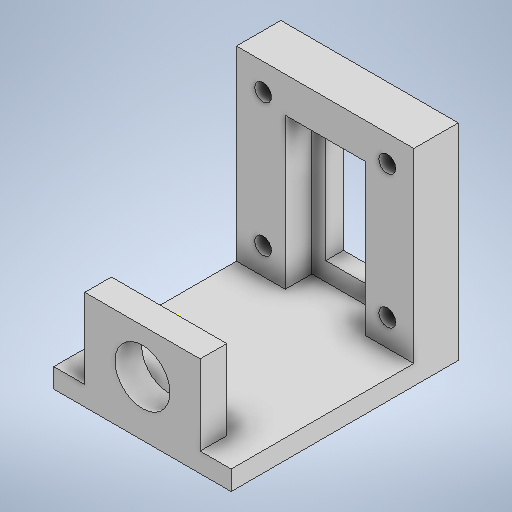
# Autodesk Inventor part: laser_krabicka2
Saved by Autodesk Inventor 2025.2 (Build 292293000, 293)
## iProperties
Created: 2025-03-31
Part Number: laser_krabicka2
Material: Všeobecné
Document SubType Name: Modeling
Designer: jakub
Density: 1 g/cm^3
Appearance: Výchozí
Author: jakub
## iProperties of the stored document laser_krabicka2_3D tisk.ipt
Created: 2025-03-31
Part Number: laser_krabicka2_3D tisk
Material: Všeobecné
Document SubType Name: Modeling
Designer: jakub
Density: 1 g/cm^3
Appearance: Výchozí
Author: jakub
Autodesk Inventor part; units mm, degrees
ref_plane "YZ Plane" through (0, 0, 0) normal (1, 0, 0) x (0, 1, 0)
ref_plane "XZ Plane" through (0, 0, 0) normal (0, 1, 0) x (-1, 0, 0)
sketch "Náčrt1" plane through (0, 0, 0) normal (0, 0, 1) x (1, 0, 0)
  line L0 (0, 12.6) -> (0, -12.6) projected
  line L1 (-12.6, 0) -> (12.6, 0) projected
  line L2 (-9, 9) -> (9, 9)
  line L3 (9, 9) -> (9, -9)
  line L4 (9, -9) -> (-9, -9)
  line L5 (-9, -9) -> (-9, 9)
  point P0 (0, 0)
  dimension "d0" = 18
  dimension "d1" = 18
  constraints: 8 end point, 2 parallel, 1 horizontal, 1 perpendicular, 2 other
  measures "d0" distance between parallel lines of L5 L3
  measures "d1" distance between parallel lines of L4 L2
extrude "Vysunutí1" add sketch "Náčrt1" against normal blind 20
sketch "Náčrt2" plane through (-9, 9, 0) normal (0, 1, 0) x (1, 0, 0)
  line L0 (18, 0) -> (0, 0) projected
  line L1 (18, 0) -> (18, 20) projected
  line L2 (0, 20) -> (18, 20) projected
  line L3 (0, 0) -> (0, 20) projected
  line L4 (1.3, 16.6) -> (1.3, 3)
  line L5 (1.3, 3) -> (16.7, 3)
  line L6 (16.7, 3) -> (16.7, 16.6)
  line L7 (16.7, 16.6) -> (1.3, 16.6)
  point P0 (9, 0)
  dimension "d4" = 3.4
  dimension "d5" = 3
  dimension "d6" = 1.3
  dimension "d7" = 1.3
  constraints: 8 end point, 3 perpendicular, 1 vertical
  measures "d4" distance between parallel lines of L2 L7
  measures "d5" distance between parallel lines of L0 L5
  measures "d6" distance between parallel lines of L6 L1
  measures "d7" distance between parallel lines of L3 L4
sketch "Náčrt3" plane through (0, 0, 0) normal (0, 0, 1) x (1, 0, 0)
  point P0 (0, 0)
extrude "Vysunutí2" cut sketch "Náčrt2" against normal blind 17 contours L7 L6 L5 L4
sketch "Náčrt4" plane through (0, 0, 0) normal (0, 0, 1) x (1, 0, 0)
  line L0 (0, 12.6) -> (0, -12.6) projected
  line L1 (-12.6, 0) -> (12.6, 0) projected
  circle A0 centre (0, -4) radius 3.1
  line L2 (-9, -9) -> (9, -9) projected
  point P0 (0, 0)
  dimension "d10" = 6.2
  dimension "d11" = 5
  constraints: 1 centre point, 1 point on line
  measures "d10" diameter of A0
  measures "d11" distance from line of L2 A0.centre
extrude "Vysunutí3" cut sketch "Náčrt4" against normal blind 3
sketch "Náčrt5" plane through (-9, 9, 0) normal (0, 1, 0) x (1, 0, 0)
  line L0 (1.3, 3) -> (1.3, 16.6) projected
  line L1 (1.3, 16.6) -> (16.7, 16.6) projected
  line L2 (16.7, 3) -> (1.3, 3) projected
  line L3 (16.7, 16.6) -> (16.7, 3) projected
  line L4 (1.3, 16.6) -> (16.7, 16.6) projected
  line L5 (1.3, 3) -> (1.3, 16.6) projected
  line L6 (16.7, 16.6) -> (16.7, 3) projected
  line L7 (16.7, 16.6) -> (16.7, 3) projected
  line L8 (16.7, 3) -> (1.3, 3) projected
  line L9 (1.3, 3) -> (1.3, 16.6) projected
  line L10 (1.3, 16.6) -> (16.7, 16.6) projected
  line L11 (18, 0) -> (0, 0) projected
  line L12 (18, 0) -> (18, 20) projected
  line L13 (0, 20) -> (18, 20) projected
  line L14 (0, 0) -> (0, 20) projected
  line L15 (1.3, 16.6) -> (0, 16.6)
  line L16 (0, 0) -> (0, 20) projected
  line L17 (0, 16.6) -> (0, 0)
  line L18 (0, 0) -> (18, 0)
  line L19 (18, 0) -> (18, 16.6)
  line L20 (18, 0) -> (18, 20) projected
  line L21 (16.7, 16.6) -> (18, 16.6)
  line L22 (16.7, 16.6) -> (16.7, 3)
  line L23 (16.7, 3) -> (1.3, 3) projected
  line L24 (16.7, 3) -> (1.3, 3)
  line L25 (1.3, 3) -> (1.3, 16.6)
  line L26 (1.3, 3) -> (1.3, 16.6)
  point P0 (9, 0)
  constraints: 18 end point, 4 point on line, 2 collinear, 2 parallel, 2 perpendicular, 1 horizontal
extrude "Vysunutí4" cut sketch "Náčrt5" against normal blind 8 contours L2 L3 L21 L12 L11 L14 L15 L0
sketch "Náčrt6" plane through (0, 0, -20) normal (0, 0, -1) x (-1, 0, 0)
  line L0 (-9, -9) -> (9, -9) projected
  line L1 (9, -9) -> (9, 9) projected
  line L2 (9, 9) -> (-9, 9) projected
  line L3 (-9, 9) -> (-9, -9) projected
  line L4 (0, -12.6) -> (0, 12.6) projected
  line L5 (-12.6, 0) -> (12.6, 0) projected
  line L6 (-2.8665, 6.0827) -> (2.9335, 6.0827)
  line L7 (2.9335, 6.0827) -> (2.9335, -5.9173)
  line L8 (2.9335, -5.9173) -> (-2.8665, -5.9173)
  line L9 (-2.8665, -5.9173) -> (-2.8665, 6.0827)
  point P0 (0, 0)
  dimension "d16" = 5.8
  dimension "d17" = 12
  constraints: 8 end point, 2 parallel, 1 horizontal, 1 perpendicular
  measures "d16" distance between parallel lines of L9 L7
  measures "d17" distance between parallel lines of L8 L6
extrude "Vysunutí5" cut sketch "Náčrt6" against normal blind 8 contours L8 L9 L5 L4 | L4 L5 L7 L8 | L9 L6 L4 L5 | L4 L6 L7 L5
sketch "Náčrt13" plane through (9, -9, -20) normal (1, 0, 0) x (0, 0, -1)
  line L0 (-3.4, 10) -> (-20, 10) projected
  line L1 (-20, 0) -> (-20, 10) projected
  line L2 (-20, 0) -> (0, 0) projected
  line L3 (0, 18) -> (0, 0) projected
  line L4 (-3.4, 18) -> (0, 18) projected
  line L5 (-3.4, 18) -> (-3.4, 10) projected
  line L6 (-3.4, 1) -> (-17, 1) projected
  line L7 (-17, 1) -> (-3.4, 1) projected
  line L8 (-17, 10) -> (-3.4, 10) projected
  line L9 (-17, 1) -> (-17, 10)
  line L10 (-17, 8.1) -> (-17, 1.9) projected
  line L11 (-3.4, 1) -> (-3.4, 10)
  line L12 (-3.4, 1) -> (-17, 1)
  line L13 (-3.4, 10) -> (-17, 10)
  point P0 (-20, 9)
  constraints: 8 end point, 3 collinear, 1 parallel
extrude "Vysunutí11" cut sketch "Náčrt13" against normal blind 20 contours L11 L6 L9 L0
sketch "Náčrt14" plane through (0, 0, 0) normal (0, 0, 1) x (1, 0, 0)
  line L0 (9, 1) -> (-9, 1) projected
  line L1 (-9, 1) -> (-9, -9) projected
  line L2 (-9, -9) -> (9, -9) projected
  line L3 (9, -9) -> (9, 1) projected
  circle A0 centre (0, -4) radius 3.1 projected
  line L4 (2.8665, -5.9173) -> (-2.9335, -5.9173) projected
  line L5 (9, -8) -> (-9, -8) projected
  line L6 (9, -8) -> (-9, -8) projected
  line L7 (9, 1) -> (6.5, 1)
  line L8 (6.5, 1) -> (6.5, -8)
  line L9 (6.5, -8) -> (9, -8)
  line L10 (9, -8) -> (9, 1)
  line L11 (-9, 1) -> (-6.5, 1)
  line L12 (-6.5, 1) -> (-6.5, -8)
  line L13 (-6.5, -8) -> (-9, -8)
  line L14 (-9, -8) -> (-9, 1)
  point P0 (0, 0)
  dimension "d44" = 2.5
  dimension "d45" = 2.5
  constraints: 16 end point, 4 parallel, 2 horizontal, 2 perpendicular, 2 point on line
  measures "d44" distance between parallel lines of L8 L10
  measures "d45" distance between parallel lines of L1 L12
extrude "Vysunutí12" cut sketch "Náčrt14" against normal blind 5 contours L3 L5 L8 L0 | L12 L5 L1 L0
sketch "Náčrt15" plane through (-9, -9, 0) normal (0, -1, 0) x (1, 0, 0)
  line L0 (0, 0) -> (18, 0) projected
  line L1 (0, 0) -> (0, -20) projected
  line L2 (18, -20) -> (0, -20) projected
  line L3 (18, 0) -> (18, -20) projected
  line L4 (18, 0) -> (0, 0)
  line L5 (0, 0) -> (0, -20)
  line L6 (0, -20) -> (18, -20)
  line L7 (18, -20) -> (18, 0)
  point P0 (9, 0)
  constraints: 8 end point, 2 parallel, 1 horizontal, 1 perpendicular
extrude "Vysunutí13" add sketch "Náčrt15" along normal blind 1.2
sketch "Náčrt16" plane through (9, -8, -16.6) normal (1, 0, 0) x (0, 0, -1)
  line L0 (0, 0) -> (-16.6, 0) projected
  line L1 (-16.6, -2.2) -> (-16.6, 0) projected
  line L2 (3.4, -2.2) -> (-16.6, -2.2) projected
  line L3 (3.4, 17) -> (3.4, -2.2) projected
  line L4 (0, 17) -> (3.4, 17) projected
  line L5 (0, 17) -> (0, 0) projected
  line L6 (-16.6, 0) -> (3.4, 0)
  line L7 (3.4, 0) -> (3.4, -2.2)
  line L8 (3.4, -2.2) -> (-16.6, -2.2)
  line L9 (-16.6, -2.2) -> (-16.6, 0)
  line L10 (0, 17) -> (3.4, 17)
  line L11 (3.4, 17) -> (3.4, 0)
  line L12 (3.4, 0) -> (0, 0)
  line L13 (0, 0) -> (0, 17)
  point P0 (-16.6, 8)
  constraints: 16 end point, 4 parallel, 2 horizontal, 2 perpendicular
extrude "Vysunutí14" add sketch "Náčrt16" along normal blind 3
sketch "Náčrt17" plane through (-9, -8, -16.6) normal (-1, 0, 0) x (0, 0, 1)
  line L0 (16.6, 0) -> (0, 0) projected
  line L1 (0, 0) -> (0, 17) projected
  line L2 (0, 17) -> (-3.4, 17) projected
  line L3 (-3.4, 17) -> (-3.4, -2.2) projected
  line L4 (16.6, -2.2) -> (-3.4, -2.2) projected
  line L5 (16.6, 0) -> (16.6, -2.2) projected
  line L6 (-3.4, 17) -> (0, 17)
  line L7 (0, 17) -> (0, -2.2)
  line L8 (0, -2.2) -> (-3.4, -2.2)
  line L9 (-3.4, -2.2) -> (-3.4, 17)
  line L10 (16.6, 0) -> (0, 0)
  line L11 (0, 0) -> (0, -2.2)
  line L12 (0, -2.2) -> (16.6, -2.2)
  line L13 (16.6, -2.2) -> (16.6, 0)
  point P0 (16.6, 8)
  point P1 (0, -1.1)
  dimension "d52" = 3.4
  constraints: 16 end point, 4 parallel, 2 horizontal, 2 perpendicular, 1 midpoint, 1 point on line
  measures "d52" distance from line of L3 point (0, -1.1)
extrude "Vysunutí15" add sketch "Náčrt17" along normal blind 3
sketch "Náčrt18" plane through (0, 0, -20) normal (0, 0, -1) x (-1, 0, 0)
  line L0 (2.9335, 6.0827) -> (2.9335, -5.9173) projected
  line L1 (2.9335, -5.9173) -> (-2.8665, -5.9173) projected
  line L2 (-2.8665, -5.9173) -> (-2.8665, 6.0827) projected
  line L3 (-2.8665, 6.0827) -> (2.9335, 6.0827) projected
  line L4 (-12, 9) -> (12, 9) projected
  line L5 (-12, -10.2) -> (-12, 9) projected
  line L6 (-12, -10.2) -> (12, -10.2) projected
  line L7 (12, 9) -> (12, -10.2) projected
  line L8 (-12, 9) -> (12, 9)
  line L9 (12, 9) -> (12, -10.2)
  line L10 (12, -10.2) -> (-12, -10.2)
  line L11 (-12, -10.2) -> (-12, 9)
  line L12 (-2.8665, 6.0827) -> (2.9335, 6.0827)
  line L13 (2.9335, 6.0827) -> (2.9335, -5.9173)
  line L14 (2.9335, -5.9173) -> (-2.8665, -5.9173)
  line L15 (-2.8665, -5.9173) -> (-2.8665, 6.0827)
  point P0 (0, 0)
  constraints: 16 end point, 4 parallel, 2 horizontal, 2 perpendicular
extrude "Vysunutí16" add sketch "Náčrt18" along normal blind 1.6
sketch "Náčrt19" plane through (12, -8, -16.6) normal (0, 0, 1) x (1, 0, 0)
  line L0 (-24, 17) -> (0, 17) projected
  line L1 (0, 0) -> (-24, 0) projected
  line L2 (-16.5, 17) -> (-7.5, 17)
  line L3 (-7.5, 17) -> (-7.5, 0)
  line L4 (-7.5, 0) -> (-16.5, 0)
  line L5 (-16.5, 0) -> (-16.5, 17)
  line L6 (-14.9335, 2.0827) -> (-14.9335, 14.0827) projected
  line L7 (-14.9335, 14.0827) -> (-9.1335, 14.0827) projected
  line L8 (-9.1335, 14.0827) -> (-9.1335, 2.0827) projected
  line L9 (-9.1335, 2.0827) -> (-14.9335, 2.0827) projected
  line L10 (0, 0) -> (-24, 0) projected
  line L11 (0, 17) -> (0, 0) projected
  line L12 (-24, 17) -> (0, 17) projected
  line L13 (-24, 0) -> (-24, 17) projected
  line L14 (-12, 17) -> (-12, 0)
  line L15 (-16.5, 17) -> (-7.5, 17)
  line L16 (-16.5, 0) -> (-7.5, 0)
  point P0 (-12, 8)
  point P1 (-16.5, 0)
  dimension "d57" = 9
  constraints: 14 end point, 2 collinear, 2 midpoint, 2 parallel, 2 point on line, 1 horizontal, 1 perpendicular, 1 other
  measures "d57" distance between parallel lines of L5 L3
ref_plane "Pracovní rovina1" through (12, -8, -9.8) normal (0, 0, 1) x (1, 0, 0)
extrude "Vysunutí17" cut sketch "Náčrt19" against normal blind 3 contours L0 L14 L7 L6 L9 L1 L5 | L0 L3 L1 L14 L9 L8 L7
sketch "Náčrt20" plane through (-12, 9, -21.6) normal (0, 1, 0) x (1, 0, 0)
  line L0 (0, -5) -> (0, 0) projected
  line L1 (24, -5) -> (24, 0) projected
  line L2 (0, 0) -> (24, 0)
  line L3 (24, 0) -> (24, -5)
  line L4 (24, -5) -> (0, -5)
  line L5 (0, -5) -> (0, 0)
  point P0 (12, -21.6)
  constraints: 8 end point, 2 parallel, 1 horizontal, 1 perpendicular
extrude "Vysunutí18" add sketch "Náčrt20" along normal blind 4
sketch "Náčrt21" plane through (4.5, -8, -16.6) normal (0, 0, 1) x (1, 0, 0)
  line L0 (0, 17) -> (0, 0) projected
  line L1 (7.5, 0) -> (0, 0) projected
  line L2 (7.5, 0) -> (7.5, 21) projected
  line L3 (-16.5, 21) -> (7.5, 21) projected
  line L4 (-16.5, 0) -> (-16.5, 21) projected
  line L5 (-9, 0) -> (-16.5, 0) projected
  line L6 (-9, 0) -> (-9, 17) projected
  line L7 (-9, 17) -> (0, 17) projected
  circle A0 centre (-11.5, 18) radius 0.95
  circle A1 centre (2.5, 3) radius 0.95
  line L8 (7.5, 10.5) -> (-16.5, 10.5)
  circle A2 centre (2.5, 18) radius 0.95
  circle A3 centre (-11.5, 3) radius 0.95
  point P0 (-4.5, 8)
  dimension "d62" = 1.9
  dimension "d63" = 3
  dimension "d64" = 5
  dimension "d65" = 1.9
  dimension "d66" = 3
  dimension "d67" = 5
  constraints: 4 centre point, 2 end point, 2 midpoint, 2 symmetric about line, 2 other
  measures "d62" diameter of A0
  measures "d63" distance from line of A0.centre L3
  measures "d64" distance from line of L4 A0.centre
  measures "d65" diameter of A1
  measures "d66" distance from line of L1 A1.centre
  measures "d67" distance from line of L2 A1.centre
extrude "Vysunutí19" cut sketch "Náčrt21" against normal up to surface (5 mm away) contours A0 | A1 | A2 | A3
sketch "Náčrt22" plane through (-12, 13, -21.6) normal (0, 1, 0) x (1, 0, 0)
  line L0 (0, 0) -> (0, -5) projected
  line L1 (0, -5) -> (24, -5) projected
  line L2 (24, -5) -> (24, 0) projected
  line L3 (24, 0) -> (0, 0) projected
  line L4 (5.5, -21.6) -> (0, -21.6) projected
  line L5 (5.5, -21.6) -> (5.5, -18.6) projected
  line L6 (18.5, -18.6) -> (5.5, -18.6) projected
  line L7 (18.5, -21.6) -> (18.5, -18.6) projected
  line L8 (18.5, -21.6) -> (24, -21.6) projected
  line L9 (24, -5) -> (24, -21.6) projected
  line L10 (24, -5) -> (16.5, -5) projected
  line L11 (16.5, -5) -> (16.5, -2) projected
  line L12 (16.5, -2) -> (7.5, -2) projected
  line L13 (7.5, -5) -> (7.5, -2) projected
  line L14 (7.5, -5) -> (0, -5) projected
  line L15 (0, -21.6) -> (0, -5) projected
  line L16 (5.5, -18.6) -> (5.5, -21.6) projected
  line L17 (18.5, -21.6) -> (5.5, -21.6) projected
  line L18 (18.5, -21.6) -> (18.5, -18.6) projected
  line L19 (18.5, -18.6) -> (5.5, -18.6) projected
  line L20 (24, 0) -> (22, 0)
  line L21 (22, 0) -> (22, -21.6)
  line L22 (22, -21.6) -> (24, -21.6)
  line L23 (24, -21.6) -> (24, 0)
  line L24 (0, 0) -> (2, 0)
  line L25 (2, 0) -> (2, -21.6)
  line L26 (2, -21.6) -> (0, -21.6)
  line L27 (0, -21.6) -> (0, 0)
  point P0 (12, -21.6)
  dimension "d71" = 2
  dimension "d72" = 2
  constraints: 16 end point, 4 parallel, 2 horizontal, 2 perpendicular, 2 point on line
  measures "d71" distance of L22.end L21.end
  measures "d72" distance of L25.end L26.end
extrude "Vysunutí20" cut sketch "Náčrt22" against normal through all contours L3 L25 L1 L0 | L1 L25 L4 L15 | L3 L2 L1 L21 | L1 L9 L8 L21
sketch "Náčrt23" plane through (0, 0, 0) normal (0, 0, 1) x (1, 0, 0)
  line L0 (10, -10.2) -> (10, -8) projected
  line L1 (6.5, -8) -> (10, -8) projected
  line L2 (6.5, -8) -> (6.5, 1) projected
  line L3 (6.5, 1) -> (-6.5, 1) projected
  line L4 (-6.5, 1) -> (-6.5, -8) projected
  line L5 (-6.5, -8) -> (-10, -8) projected
  line L6 (-10, -8) -> (-10, -10.2) projected
  line L7 (-10, -10.2) -> (10, -10.2) projected
  circle A0 centre (0, -4) radius 3.1 projected
  line L8 (-10, -8) -> (10, -8)
  line L9 (10, -8) -> (10, -10.2)
  line L10 (10, -10.2) -> (-10, -10.2)
  line L11 (-10, -10.2) -> (-10, -8)
  point P0 (0, 0)
  constraints: 8 end point, 2 parallel, 1 horizontal, 1 perpendicular
extrude "Vysunutí21" add sketch "Náčrt23" along normal blind 4 contours L7 L6 L5 L8 L1 L0
sketch "Náčrt24" plane through (-9, -8, 0) normal (0, 1, 0) x (1, 0, 0)
  line L0 (2.5, 3) -> (2.5, 0) projected
  line L1 (15.5, 0) -> (2.5, 0) projected
  line L2 (15.5, 0) -> (15.5, 3) projected
  line L3 (15.5, 3) -> (2.5, 3) projected
  line L4 (2.5, 0) -> (2.5, 3) projected
  line L5 (15.5, 3) -> (2.5, 3) projected
  line L6 (15.5, 0) -> (15.5, 3) projected
  line L7 (2.5, 0) -> (15.5, 0) projected
  line L8 (-1, 16.6) -> (-1, -4) projected
  line L9 (19, -4) -> (-1, -4) projected
  line L10 (19, -4) -> (19, 16.6) projected
  line L11 (19, 16.6) -> (13.5, 16.6) projected
  line L12 (13.5, 16.6) -> (13.5, 19.6) projected
  line L13 (13.5, 19.6) -> (4.5, 19.6) projected
  line L14 (4.5, 16.6) -> (4.5, 19.6) projected
  line L15 (4.5, 16.6) -> (-1, 16.6) projected
  line L16 (15.5, 3) -> (2.5, 3) projected
  line L17 (2.5, 3) -> (2.5, 0) projected
  line L18 (2.5, -1) -> (15.5, -1)
  line L19 (15.5, -1) -> (15.5, -4)
  line L20 (15.5, -4) -> (2.5, -4)
  line L21 (2.5, -4) -> (2.5, -1)
  line L22 (11.8665, 21.6) -> (6.0665, 21.6) projected
  point P0 (9, 0)
  point P1 (15.5, -2.5)
  point P2 (2.5, -4)
  dimension "d77" = 3
  dimension "d78" = 13
  dimension "d87" = 3.5
  constraints: 8 end point, 2 parallel, 1 horizontal, 1 midpoint, 1 perpendicular, 1 point on line
  measures "d77" distance between parallel lines of L20 L18
  measures "d78" distance from line of point (15.5, -2.5) L21
  measures "d87" distance between parallel lines of L10 L19
extrude "Vysunutí22" add sketch "Náčrt24" along normal up to surface (9 mm away) contours L21 L18 L19 L9
sketch "Náčrt25" plane through (0, 0, 4) normal (0, 0, 1) x (1, 0, 0)
  line L0 (10, -8) -> (6.5, -8) projected
  line L1 (6.5, -8) -> (6.5, 1) projected
  line L2 (-6.5, 1) -> (6.5, 1) projected
  line L3 (-6.5, -8) -> (-6.5, 1) projected
  line L4 (-6.5, -8) -> (-10, -8) projected
  line L5 (-10, -8) -> (-10, -10.2) projected
  line L6 (-10, -10.2) -> (10, -10.2) projected
  line L7 (10, -10.2) -> (10, -8) projected
  circle A0 centre (0, -4) radius 3.1 projected
  circle A1 centre (0, -4) radius 3.1
  point P0 (0, 0)
  constraints: 1 centre point, 1 coincident, 1 concentric
extrude "Vysunutí23" cut sketch "Náčrt25" against normal blind 10 contours A0
sketch "Náčrt26" plane through (-9, 1, 0) normal (0, 1, 0) x (1, 0, 0)
  line L0 (2.5, 3) -> (2.5, 0) projected
  line L1 (15.5, 0) -> (2.5, 0) projected
  line L2 (15.5, 0) -> (15.5, 3) projected
  line L3 (15.5, 3) -> (2.5, 3) projected
  line L4 (2.5, 3) -> (15.5, 3)
  line L5 (15.5, 3) -> (15.5, 0)
  line L6 (15.5, 0) -> (2.5, 0)
  line L7 (2.5, 0) -> (2.5, 3)
  line L8 (2.5, 3) -> (15.5, 3)
  line L9 (15.5, 3) -> (15.5, 0)
  line L10 (15.5, 0) -> (2.5, 0)
  line L11 (2.5, 0) -> (2.5, 3)
  point P0 (9, 0)
  constraints: 16 end point, 4 parallel, 2 horizontal, 2 perpendicular
extrude "Vysunutí24" cut sketch "Náčrt26" against normal up to surface (9 mm away)
